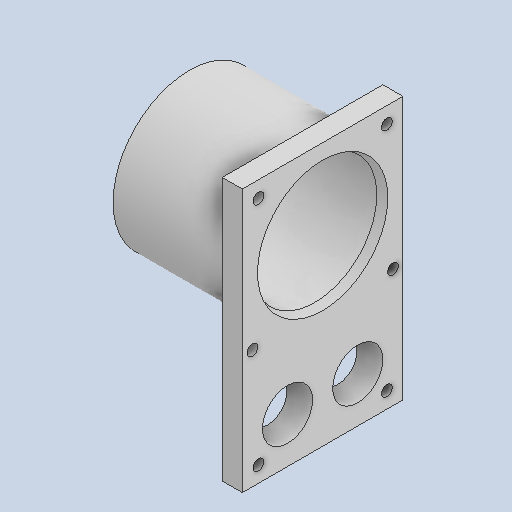
# Autodesk Inventor part: Engine Head Bottom
Saved by Autodesk Inventor 2023 (Build 270158000, 158)
## iProperties
Created: 2022-12-23
Part Number: Engine Head Bottom
Material: Generic
Document SubType Name: Modeling
Designer: tgr41
Density: 1 g/cm^3
Appearance: Default
Author: tgr41
Autodesk Inventor part; units mm, degrees
ref_plane "YZ Plane" through (0, 0, 0) normal (1, 0, 0) x (0, 1, 0)
ref_plane "XZ Plane" through (0, 0, 0) normal (0, 1, 0) x (-1, 0, 0)
ref_plane "XY Plane" through (0, 0, 0) normal (0, 0, 1) x (1, 0, 0)
sketch "Sketch1" plane through (0, 0, 0) normal (1, 0, 0) x (0, 1, 0)
  line L0 (0, 0) -> (83.185, 0)
  line L1 (83.185, 0) -> (83.185, -50.8)
  line L2 (83.185, -50.8) -> (0, -50.8)
  line L3 (0, -50.8) -> (0, 0)
  circle A0 centre (57.785, -25.4) radius 19.685
  circle A1 centre (14.2875, -14.2875) radius 7.9375
  circle A2 centre (14.2875, -36.5125) radius 7.9375
  circle A3 centre (5.08, -5.08) radius 1.7145
  circle A4 centre (5.08, -45.72) radius 1.7145
  circle A5 centre (78.105, -5.08) radius 1.7145
  circle A6 centre (78.105, -45.72) radius 1.7145
  line L4 (83.185, 0) -> (32.385, 0)
  circle A7 centre (37.465, -47.625) radius 1.7145
  circle A8 centre (37.465, -3.175) radius 1.7145
  circle A9 centre (57.785, -25.4) radius 24.13
  dimension "d0" = 83.185
  dimension "d1" = 50.8
  dimension "d2" = 39.37
  dimension "d3" = 25.4
  dimension "d4" = 25.4
  dimension "d5" = 15.875
  dimension "d6" = 15.875
  dimension "d7" = 14.2875
  dimension "d8" = 14.2875
  dimension "d9" = 14.2875
  dimension "d10" = 14.2875
  dimension "d16" = 3.429
  dimension "d17" = 5.08
  dimension "d18" = 5.08
  dimension "d19" = 50.8
  dimension "d20" = 3.429
  dimension "d21" = 3.175
  dimension "d23" = 48.26
  dimension "d32" = 5.08
  dimension "d33" = 5.08
  dimension "d34" = 3.175
  dimension "d35" = 5.08
  dimension "d36" = 5.08
  dimension "d37" = 5.08
  dimension "d38" = 5.08
  constraints: 10 centre point, 10 end point, 2 parallel, 1 coincident, 1 horizontal, 1 perpendicular, 1 point on line
  measures "d0" distance of L1.end L2.end
  measures "d1" distance of L0.end L1.end
  measures "d2" diameter of A0
  measures "d3" distance from line of L1 A0.centre
  measures "d4" distance from line of L2 A0.centre
  measures "d5" diameter of A1
  measures "d6" diameter of A2
  measures "d7" distance from line of L3 A1.centre
  measures "d8" distance from line of L3 A2.centre
  measures "d9" distance from line of L2 A2.centre
  measures "d10" distance from line of L0 A1.centre
  measures "d16" diameter of A3
  measures "d17" distance from line of L3 A3.centre
  measures "d18" distance from line of L0 A3.centre
  measures "d19" distance of L0.end L4.end
  measures "d20" diameter of A7
  measures "d21" distance from line of L2 A7.centre
  measures "d23" diameter of A9
  measures "d32" distance from line of L2 A4.centre
  measures "d33" distance from line of L3 A4.centre
  measures "d34" distance from line of L0 A8.centre
  measures "d35" distance from line of L2 A6.centre
  measures "d36" distance from line of L1 A6.centre
  measures "d37" distance from line of L1 A5.centre
  measures "d38" distance from line of L4 A5.centre
extrude "Extrusion1" add sketch "Sketch1" along normal blind 6.35 contours L0 L1 L2 L3 | A9
draft "FaceDraft1" angle 16 pull direction (1, 0, 0) faces at (4.2333, 22.1993, -37.1512) (4.2333, 22.1993, -14.9262) fixed edges at (6.35, 6.35, -36.5125) (6.35, 6.35, -14.2875)
extrude "Extrusion2" add sketch "Sketch1" against normal blind 35.814 contours A9
chamfer "Chamfer1" distance 2.54 angle 20 1 edges at (6.35, 38.1, -25.4) measured on face at (-7.7047, 77.4062, -26.984)
chamfer "Chamfer2" distance 2.54 angle 20 1 edges at (-35.814, 38.1, -25.4) measured on face at (-9.398, 77.2151, -28.5577)
body "Solid1"
